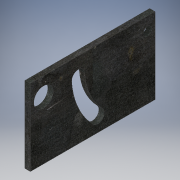
# Autodesk Inventor part: side_plate
Saved by Autodesk Inventor 2017 (Build 210142000, 142)
## iProperties
Created: 2017-01-16
Part Number: side_plate
Material: Steel
Document SubType Name: Modeling
Designer: mmarkle
Density: 7.85 g/cm^3
Appearance: Plate
Mass: 1109.75 g
Surface Area: 429.146 cm^2
Volume: 141.369 cm^3
Author: mmarkle
Autodesk Inventor part; units mm, degrees
ref_plane "YZ Plane" through (0, 0, 0) normal (1, 0, 0) x (0, 1, 0)
ref_plane "XZ Plane" through (0, 0, 0) normal (0, 1, 0) x (-1, 0, 0)
ref_plane "XY Plane" through (0, 0, 0) normal (0, 0, 1) x (1, 0, 0)
sketch "Sketch1" plane through (0, 0, 0) normal (1, 0, 0) x (0, 1, 0)
  line L0 (-55.5791, 90.9825) -> (55.5791, 90.9825)
  line L1 (55.5791, 90.9825) -> (55.5791, -90.9825)
  line L2 (55.5791, -90.9825) -> (-55.5791, -90.9825)
  line L3 (-55.5791, -90.9825) -> (-55.5791, 90.9825)
  line L4 (-55.5791, 90.9825) -> (55.5791, -90.9825) construction
  line L5 (55.5791, 90.9825) -> (-55.5791, -90.9825) construction
  circle A0 centre (35.8863, -80.1209) radius 6.35
  arc A1 (28.845, 21.2348) -> (-35.1241, -7.4567) centre (35.8863, -80.1209) ccw construction
  arc A2 (28.1849, 30.7369) -> (-41.7813, -0.6445) centre (35.8863, -80.1209) ccw
  arc A3 (29.5052, 11.7327) -> (-28.4669, -14.269) centre (35.8863, -80.1209) ccw
  arc A4 (29.5052, 11.7327) -> (28.1849, 30.7369) centre (28.845, 21.2348) ccw
  arc A5 (-41.7813, -0.6445) -> (-28.4669, -14.269) centre (-35.1241, -7.4567) ccw
  circle A6 centre (28.845, 71.7808) radius 14.2875
  point P0 (0, 0)
  dimension "d2" = 12.7
  dimension "d3" = 101.6
  dimension "d4" = 19.05
  dimension "d5" = 28.575
  dimension "d9" = 50.546
  dimension "d10" = 0
  dimension "d11" = 181.965
  dimension "d12" = 111.1583
  constraints: 12 end point, 10 point on circle, 7 centre point, 4 tangent, 2 midpoint, 2 parallel, 1 coincident, 1 horizontal, 1 perpendicular
  measures "d2" diameter of A0
  measures "d3" radius of A1
  measures "d4" diameter of A4
  measures "d5" diameter of A6
  measures "d9" distance of A6.centre A1.start
  measures "d10" horizontal distance of A6.centre A1.start
  measures "d11" distance of L0.end L1.end
  measures "d12" distance of L0.start L0.end
extrude "Extrusion1" add sketch "Sketch1" along normal blind 7.9375
body "Solid1"
